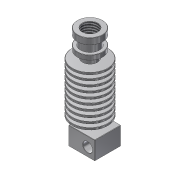
# Autodesk Inventor part: Extruder Heat Sink
Saved by Autodesk Inventor 2015 (Build 190159000, 159)
## iProperties
Created: 2019-05-04
Part Number: Extruder Heat Sink
Material: Aluminum 6061-AHC
Document SubType Name: Modeling
Designer: Workshop
Density: 2.7 g/cm^3
Appearance: Aluminum - Dark
Author: Workshop
Autodesk Inventor part; units mm, degrees
ref_plane "YZ Plane" through (0, 0, 0) normal (1, 0, 0) x (0, 1, 0)
ref_plane "XZ Plane" through (0, 0, 0) normal (0, 1, 0) x (-1, 0, 0)
ref_plane "XY Plane" through (0, 0, 0) normal (0, 0, 1) x (1, 0, 0)
sketch "Sketch1" plane through (0, 0, 0) normal (0, 0, 1) x (1, 0, 0)
  circle A0 centre (0, 0) radius 8
  dimension "d0" = 16
  constraints: 1 centre point, 1 coincident
  measures "d0" diameter of A0
extrude "Extrusion1" add sketch "Sketch1" against normal blind 4
sketch "Sketch2" plane through (0, 0, -4) normal (0, 0, -1) x (-1, 0, 0)
  circle A0 centre (0, 0) radius 6
  dimension "d3" = 12
  constraints: 1 centre point, 1 coincident
  measures "d3" diameter of A0
extrude "Extrusion2" add sketch "Sketch2" along normal blind 5.4
sketch "Sketch3" plane through (0, 0, -9.4) normal (0, 0, -1) x (-1, 0, 0)
  circle A0 centre (0, 0) radius 8
  circle A1 centre (0, 0) radius 8 projected
  constraints: 1 centre point, 1 coincident, 1 concentric
extrude "Extrusion3" add sketch "Sketch3" along normal blind 3
sketch "Sketch4" plane through (0, 0, -12.4) normal (0, 0, -1) x (-1, 0, 0)
  circle A0 centre (0, 0) radius 4.7
  dimension "d8" = 9.4
  constraints: 1 centre point, 1 coincident
  measures "d8" diameter of A0
extrude "Extrusion4" add sketch "Sketch4" along normal blind 4.32
sketch "Sketch5" plane through (0, 0, -16.72) normal (0, 0, -1) x (-1, 0, 0)
  circle A0 centre (0, 0) radius 11.25
  dimension "d11" = 22.5
  constraints: 1 centre point, 1 coincident
  measures "d11" diameter of A0
extrude "Extrusion5" add sketch "Sketch5" along normal blind 1.35
sketch "Sketch6" plane through (0, 0, -18.07) normal (0, 0, -1) x (-1, 0, 0)
  circle A0 centre (0, 0) radius 4.7
  constraints: 1 centre point, 1 coincident
extrude "Extrusion6" add sketch "Sketch6" along normal blind 2
sketch "Sketch7" plane through (0, 0, -20.07) normal (0, 0, -1) x (-1, 0, 0)
  circle A0 centre (0, 0) radius 11.25
  circle A1 centre (0, 0) radius 11.25 projected
  constraints: 1 centre point, 1 coincident, 1 concentric
extrude "Extrusion7" add sketch "Sketch7" along normal blind 1.35
sketch "Sketch8" plane through (0, 0, -21.42) normal (0, 0, -1) x (-1, 0, 0)
  circle A0 centre (0, 0) radius 4.7
  constraints: 1 centre point, 1 coincident
extrude "Extrusion8" add sketch "Sketch8" along normal blind 2
sketch "Sketch9" plane through (0, 0, -23.42) normal (0, 0, -1) x (-1, 0, 0)
  circle A0 centre (0, 0) radius 11.25
  circle A1 centre (0, 0) radius 11.25 projected
  constraints: 1 centre point, 1 coincident, 1 concentric
extrude "Extrusion9" add sketch "Sketch9" along normal blind 1.35
sketch "Sketch10" plane through (0, 0, -24.77) normal (0, 0, -1) x (-1, 0, 0)
  circle A0 centre (0, 0) radius 4.7
  constraints: 1 centre point, 1 coincident
extrude "Extrusion10" add sketch "Sketch10" along normal blind 2
sketch "Sketch11" plane through (0, 0, -26.77) normal (0, 0, -1) x (-1, 0, 0)
  circle A0 centre (0, 0) radius 11.25
  circle A1 centre (0, 0) radius 11.25 projected
  constraints: 1 centre point, 1 coincident, 1 concentric
extrude "Extrusion11" add sketch "Sketch11" along normal blind 1.35
sketch "Sketch12" plane through (0, 0, -28.12) normal (0, 0, -1) x (-1, 0, 0)
  circle A0 centre (0, 0) radius 4.7
  constraints: 1 centre point, 1 coincident
extrude "Extrusion12" add sketch "Sketch12" along normal blind 2
sketch "Sketch13" plane through (0, 0, -30.12) normal (0, 0, -1) x (-1, 0, 0)
  circle A0 centre (0, 0) radius 11.25
  circle A1 centre (0, 0) radius 11.25 projected
  constraints: 1 centre point, 1 coincident, 1 concentric
extrude "Extrusion13" add sketch "Sketch13" along normal blind 1.35
sketch "Sketch14" plane through (0, 0, -31.47) normal (0, 0, -1) x (-1, 0, 0)
  circle A0 centre (0, 0) radius 4.7
  constraints: 1 centre point, 1 coincident
extrude "Extrusion14" add sketch "Sketch14" along normal blind 2
sketch "Sketch15" plane through (0, 0, -33.47) normal (0, 0, -1) x (-1, 0, 0)
  circle A0 centre (0, 0) radius 11.25
  circle A1 centre (0, 0) radius 11.25 projected
  constraints: 1 centre point, 1 coincident, 1 concentric
extrude "Extrusion15" add sketch "Sketch15" along normal blind 1.35
sketch "Sketch16" plane through (0, 0, -34.82) normal (0, 0, -1) x (-1, 0, 0)
  circle A0 centre (0, 0) radius 4.7
  constraints: 1 centre point, 1 coincident
extrude "Extrusion16" add sketch "Sketch16" along normal blind 2
sketch "Sketch17" plane through (0, 0, -36.82) normal (0, 0, -1) x (-1, 0, 0)
  circle A0 centre (0, 0) radius 11.25
  circle A1 centre (0, 0) radius 11.25 projected
  constraints: 1 centre point, 1 coincident, 1 concentric
extrude "Extrusion17" add sketch "Sketch17" along normal blind 1.35
sketch "Sketch18" plane through (0, 0, -38.17) normal (0, 0, -1) x (-1, 0, 0)
  circle A0 centre (0, 0) radius 4.7
  constraints: 1 centre point, 1 coincident
extrude "Extrusion18" add sketch "Sketch18" along normal blind 2
sketch "Sketch19" plane through (0, 0, -40.17) normal (0, 0, -1) x (-1, 0, 0)
  circle A0 centre (0, 0) radius 11.25
  circle A1 centre (0, 0) radius 11.25 projected
  constraints: 1 centre point, 1 coincident, 1 concentric
extrude "Extrusion19" add sketch "Sketch19" along normal blind 1.35
sketch "Sketch20" plane through (0, 0, -41.52) normal (0, 0, -1) x (-1, 0, 0)
  circle A0 centre (0, 0) radius 4.7
  constraints: 1 centre point, 1 coincident
extrude "Extrusion20" add sketch "Sketch20" along normal blind 2
sketch "Sketch21" plane through (0, 0, -43.52) normal (0, 0, -1) x (-1, 0, 0)
  circle A0 centre (0, 0) radius 11.25
  circle A1 centre (0, 0) radius 11.25 projected
  constraints: 1 centre point, 1 coincident, 1 concentric
extrude "Extrusion21" add sketch "Sketch21" along normal blind 1.35
sketch "Sketch22" plane through (0, 0, -44.87) normal (0, 0, -1) x (-1, 0, 0)
  circle A0 centre (0, 0) radius 4.7
  constraints: 1 centre point, 1 coincident
extrude "Extrusion22" add sketch "Sketch22" along normal blind 2
sketch "Sketch23" plane through (0, 0, -46.87) normal (0, 0, -1) x (-1, 0, 0)
  circle A0 centre (0, 0) radius 11.25
  circle A1 centre (0, 0) radius 11.25 projected
  constraints: 1 centre point, 1 coincident, 1 concentric
extrude "Extrusion23" add sketch "Sketch23" along normal blind 1.35
sketch "Sketch24" plane through (0, 0, -48.22) normal (0, 0, -1) x (-1, 0, 0)
  circle A0 centre (0, 0) radius 3
  dimension "d50" = 6
  constraints: 1 centre point, 1 coincident
  measures "d50" diameter of A0
extrude "Extrusion24" add sketch "Sketch24" along normal blind 3.6
sketch "Sketch25" plane through (0, 0, -51.82) normal (0, 0, -1) x (-1, 0, 0)
  line L0 (5.25, -8.25) -> (-11.25, -8.25)
  line L1 (-11.25, -8.25) -> (-11.25, 8.25)
  line L2 (-11.25, 8.25) -> (5.25, 8.25)
  line L3 (5.25, 8.25) -> (5.25, -8.25)
  circle A0 centre (0, 0) radius 11.25 projected
  point P0 (5.25, 0)
  dimension "d53" = 16.5
  dimension "d54" = 16.5
  constraints: 8 end point, 2 parallel, 1 horizontal, 1 horizontal alignment, 1 midpoint, 1 perpendicular, 1 tangent
  measures "d53" distance of L1.end L2.end
  measures "d54" distance of L0.end L1.end
extrude "Extrusion25" add sketch "Sketch25" along normal blind 11.5 contours L0 A0 L2 L3 | L0 L1 A0 | L1 L2 A0 picked at (-0.25, 0)
sketch "Sketch26" plane through (0, 0, -63.32) normal (0, 0, -1) x (-1, 0, 0)
  circle A0 centre (0, 0) radius 3 projected
  line L0 (-4, -2.3094) -> (-4, 2.3094)
  line L1 (-4, 2.3094) -> (0, 4.6188)
  line L2 (0, 4.6188) -> (4, 2.3094)
  line L3 (4, 2.3094) -> (4, -2.3094)
  line L4 (4, -2.3094) -> (0, -4.6188)
  line L5 (0, -4.6188) -> (-4, -2.3094)
  line L6 (5.25, -8.25) -> (5.25, 8.25) projected
  dimension "d58" = 8
  constraints: 12 end point, 1 coincident, 1 parallel, 13 other
  measures "d58" distance between parallel lines of L0 L3
extrude "Extrusion26" add sketch "Sketch26" along normal blind 5 contours A0 | L0 L1 L2 L3 L4 L5
chamfer "Chamfer1" distance 3.7 angle 45 6 edges at (-4, 0, -68.32) (-2, 3.4641, -68.32) (2, 3.4641, -68.32) (4, 0, -68.32) (2, -3.4641, -68.32) (-2, -3.4641, -68.32)
sketch "Sketch27" plane through (0, 0, -68.32) normal (0, 0, -1) x (-1, 0, 0)
  circle A0 centre (0, 0) radius 0.2
  dimension "d64" = 0.4
  constraints: 1 centre point, 1 coincident
  measures "d64" diameter of A0
extrude "Extrusion27" cut sketch "Sketch27" against normal blind 75.75
sketch "Sketch28" plane through (0, 0, 0) normal (0, 0, 1) x (1, 0, 0)
  circle A0 centre (0, 0) radius 1
  dimension "d67" = 2
  constraints: 1 centre point, 1 coincident
  measures "d67" diameter of A0
extrude "Extrusion28" cut sketch "Sketch28" against normal blind 61.5
sketch "Sketch29" plane through (0, 0, 0) normal (0, 0, 1) x (1, 0, 0)
  circle A0 centre (0, 0) radius 0.2 projected
  circle A1 centre (0, 0) radius 4.75
  dimension "d70" = 9.5
  constraints: 1 centre point, 1 coincident
  measures "d70" diameter of A1
extrude "Extrusion29" cut sketch "Sketch29" against normal blind 8 contours A0 | A1
chamfer "Chamfer2" distance 3.75 angle 45 1 edges at (-1, 0, -8)
thread "Thread1" size "M10x1.5" class "6H" standard "ANSI Metric M Profile" full length
chamfer "Chamfer3" distance 0.2 angle 45 25 edges at (-8, 0, 0) (-8, 0, -4) (8, 0, -9.4) (8, 0, -12.4) (-4.75, 0, 0) (11.25, 0, -16.72) (11.25, 0, -18.07) (11.25, 0, -20.07) (11.25, 0, -21.42) (11.25, 0, -23.42) (11.25, 0, -24.77) (11.25, 0, -26.77) (11.25, 0, -28.12) (11.25, 0, -30.12) (11.25, 0, -31.47) (11.25, 0, -33.47) (11.25, 0, -34.82) (11.25, 0, -36.82) (11.25, 0, -38.17) (11.25, 0, -40.17) (11.25, 0, -41.52) (11.25, 0, -43.52) (11.25, 0, -44.87) (11.25, 0, -46.87) (11.25, 0, -48.22)
chamfer "Chamfer4" distance 0.2 angle 45 4 edges at (-5.25, -8.25, -57.57) (11.25, -8.25, -57.57) (-5.25, 8.25, -57.57) (11.25, 8.25, -57.57)
thread "Thread2" size "M6x1" class "6g" standard "ANSI Metric M Profile" full length
sketch "Sketch30" plane through (-5.05, 8.25, -51.82) normal (0, 1, 0) x (1, 0, 0)
  circle A0 centre (11.8, 6.0984) radius 3
  line L0 (16.3, 0) -> (16.3, 11.5) projected
  point P0 (5.05, -51.82)
  dimension "d86" = 6
  dimension "d87" = 4.5
  constraints: 1 centre point
  measures "d86" diameter of A0
  measures "d87" distance from line of L0 A0.centre
extrude "Extrusion30" cut sketch "Sketch30" against normal blind 16.5
chamfer "Chamfer5" distance 0.2 angle 45 2 edges at (3.75, -8.25, -57.9184) (3.75, 8.25, -57.9184)
chamfer "Chamfer6" distance 0.2 angle 45 16 edges at (3, -8.25, -51.82) (11.25, 0, -51.82) (3, 8.25, -51.82) (-5.25, 0, -51.82) (-5.15, -8.15, -51.82) (11.15, -8.15, -51.82) (11.15, 8.15, -51.82) (-5.15, 8.15, -51.82) (-5.15, 8.15, -63.32) (-5.15, -8.15, -63.32) (11.15, -8.15, -63.32) (11.15, 8.15, -63.32) (3, 8.25, -63.32) (11.25, 0, -63.32) (3, -8.25, -63.32) (-5.25, 0, -63.32)
body "Solid1"
